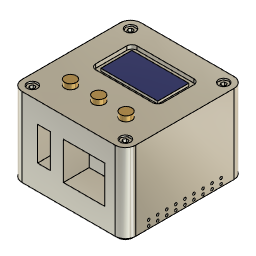
NanoPi v2 v1 (Autodesk Fusion 360 design; units mm, degrees)
Autodesk Fusion 360 part; units mm, degrees
sketch "草图1" plane through (0, 0, 0) normal (0, 0, 1) x (1, 0, 0)
  line L0 (4, 0) -> (40, 0)
  line L1 (44, 4) -> (44, 42)
  line L2 (40, 46) -> (4, 46)
  line L3 (0, 42) -> (0, 4)
  arc A0 (4, 46) -> (0, 42) centre (4, 42) ccw
  arc A1 (44, 42) -> (40, 46) centre (40, 42) ccw
  arc A2 (40, 0) -> (44, 4) centre (40, 4) ccw
  arc A3 (0, 4) -> (4, 0) centre (4, 4) ccw
  point P0 (44, 0)
  point P1 (0, 46)
  dimension "d1" = 44
  dimension "d2" = 46
  dimension "d3" = 4
  dimension "d4" = 4
  dimension "d5" = 4
  dimension "d6" = 4
  constraint horizontal L0
  constraint vertical L1
  constraint horizontal L2
  constraint vertical L3
  constraint coincident P1 L2
  constraint coincident P1 L3
  constraint tangent L2 A0
  constraint tangent L3 A0
  constraint tangent L2 A1
  constraint tangent L1 A1
  constraint coincident P0 L1
  constraint coincident P0 L0
  constraint tangent L1 A2
  constraint tangent L0 A2
  constraint coincident origin L3
  constraint coincident origin L0
  constraint tangent L3 A3
  constraint tangent L0 A3
  measures "d1" distance of origin P0
  measures "d2" distance of origin P1
  measures "d3" radius of A0
  measures "d4" radius of A1
  measures "d5" radius of A2
  measures "d6" radius of A3
extrude "拉伸1" add sketch "草图1" along normal blind 30.5 makes body 1
sketch "草图2" plane through (0, 0, 30.5) normal (0, 0, 1) x (-1, 0, 0)
  arc A0 (0, -4) -> (-4, 0) centre (-4, -4) ccw
  line L0 (-4, 0) -> (-40, 0)
  arc A1 (-40, 0) -> (-44, -4) centre (-40, -4) ccw
  line L1 (-44, -4) -> (-44, -42)
  arc A2 (-44, -42) -> (-40, -46) centre (-40, -42) ccw
  line L2 (-40, -46) -> (-4, -46)
  arc A3 (-4, -46) -> (0, -42) centre (-4, -42) ccw
  line L3 (0, -42) -> (0, -4)
  line L4 (-11, -37.5) -> (-33, -37.5)
  line L5 (-35, -35.5) -> (-35, -23.5)
  line L6 (-33, -21.5) -> (-11, -21.5)
  line L7 (-9, -23.5) -> (-9, -35.5)
  arc A4 (-11, -37.5) -> (-9, -35.5) centre (-11, -35.5) ccw
  arc A5 (-35, -35.5) -> (-33, -37.5) centre (-33, -35.5) ccw
  arc A6 (-33, -21.5) -> (-35, -23.5) centre (-33, -23.5) ccw
  arc A7 (-9, -23.5) -> (-11, -21.5) centre (-11, -23.5) ccw
  point P0 (-9, -37.5)
  point P1 (-35, -37.5)
  point P2 (-9, -21.5)
  dimension "d9" = 26
  dimension "d10" = 16
  dimension "d11" = 8.5
  dimension "d12" = 9
  dimension "d13" = 2
  dimension "d14" = 2
  dimension "d15" = 2
  dimension "d16" = 2
  constraint horizontal L4
  constraint vertical L5
  constraint horizontal L6
  constraint vertical L7
  constraint coincident P0 L4
  constraint coincident P0 L7
  constraint tangent L4 A4
  constraint tangent L7 A4
  constraint coincident P1 L4
  constraint coincident P1 L5
  constraint tangent L4 A5
  constraint tangent L5 A5
  constraint tangent L5 A6
  constraint tangent L6 A6
  constraint coincident P2 L7
  constraint coincident P2 L6
  constraint tangent L7 A7
  constraint tangent L6 A7
  measures "d9" distance of P0 P1
  measures "d10" distance of P0 P2
  measures "d11" distance of L2 L4
  measures "d12" distance of L3 L7
  measures "d13" radius of A4
  measures "d14" radius of A5
  measures "d15" radius of A6
  measures "d16" radius of A7
extrude "拉伸2" cut sketch "草图2" against normal blind 1.5 contours L4 L5 L6 L7 A4 A5 A6 A7 bodies 1
sketch "草图3" plane through (0, 0, 29) normal (0, 0, 1) x (-1, 0, 0)
  arc A0 (-11, -37.5) -> (-9, -35.5) centre (-11, -35.5) ccw
  line L0 (-9, -35.5) -> (-9, -23.5)
  arc A1 (-9, -23.5) -> (-11, -21.5) centre (-11, -23.5) ccw
  line L1 (-11, -21.5) -> (-33, -21.5)
  arc A2 (-33, -21.5) -> (-35, -23.5) centre (-33, -23.5) ccw
  line L2 (-35, -23.5) -> (-35, -35.5)
  arc A3 (-35, -35.5) -> (-33, -37.5) centre (-33, -35.5) ccw
  line L3 (-33, -37.5) -> (-11, -37.5)
  line L4 (-11, -35.5) -> (-33, -35.5)
  line L5 (-33, -35.5) -> (-33, -23.5)
  line L6 (-33, -23.5) -> (-11, -23.5)
  line L7 (-11, -23.5) -> (-11, -35.5)
  constraint horizontal L4
  constraint vertical L5
  constraint horizontal L6
  constraint vertical L7
  constraint coincident A2.centre L5.end
  constraint coincident A0.centre L4.start
extrude "拉伸3" add sketch "草图3" along normal blind 1 contours L4 L5 L6 L7 bodies 1
sketch "草图4" plane through (0, 0, 30.5) normal (0, 0, 1) x (-1, 0, 0)
  line L0 (-9, -23.5) -> (-9, -35.5)
  arc A0 (-11, -37.5) -> (-9, -35.5) centre (-11, -35.5) ccw
  line L1 (-11, -37.5) -> (-33, -37.5)
  arc A1 (-35, -35.5) -> (-33, -37.5) centre (-33, -35.5) ccw
  line L2 (-35, -35.5) -> (-35, -23.5)
  arc A2 (-33, -21.5) -> (-35, -23.5) centre (-33, -23.5) ccw
  line L3 (-33, -21.5) -> (-11, -21.5)
  arc A3 (-9, -23.5) -> (-11, -21.5) centre (-11, -23.5) ccw
  arc A4 (0, -4) -> (-4, 0) centre (-4, -4) ccw
  line L4 (-4, 0) -> (-40, 0)
  arc A5 (-40, 0) -> (-44, -4) centre (-40, -4) ccw
  line L5 (-44, -4) -> (-44, -42)
  arc A6 (-44, -42) -> (-40, -46) centre (-40, -42) ccw
  line L6 (-40, -46) -> (-4, -46)
  arc A7 (-4, -46) -> (0, -42) centre (-4, -42) ccw
  line L7 (0, -42) -> (0, -4)
  circle A8 centre (-4, -42) radius 2
  circle A9 centre (-40, -42) radius 2
  circle A10 centre (-4, -4) radius 2
  circle A11 centre (-40, -4) radius 2
  dimension "d21" = 4
  dimension "d22" = 4
  dimension "d23" = 4
  dimension "d24" = 4
  constraint concentric A7 A8
  constraint concentric A6 A9
  constraint concentric A4 A10
  constraint concentric A5 A11
  measures "d21" diameter of A8
  measures "d22" diameter of A9
  measures "d23" diameter of A10
  measures "d24" diameter of A11
extrude "拉伸4" cut sketch "草图4" against normal blind 2 contours A8 | A9 | A10 | A11 bodies 1
sketch "草图5" plane through (0, 0, 28.5) normal (0, 0, 1) x (-1, 0, 0)
  circle A0 centre (-4, -42) radius 2
  line L0 (-4.9596, -43.7548) -> (-2.9601, -43.7084)
  line L1 (-2.9601, -43.7084) -> (-2.0005, -41.9537)
  line L2 (-2.0005, -41.9537) -> (-3.0404, -40.2452)
  line L3 (-3.0404, -40.2452) -> (-5.0399, -40.2916)
  line L4 (-5.0399, -40.2916) -> (-5.9995, -42.0463)
  line L5 (-5.9995, -42.0463) -> (-4.9596, -43.7548)
  line L6 (-4.5137, -42.8579) -> (-3.5139, -42.8739)
  line L7 (-3.5139, -42.8739) -> (-3.0001, -42.016)
  line L8 (-3.0001, -42.016) -> (-3.4863, -41.1421)
  line L9 (-3.4863, -41.1421) -> (-4.4861, -41.1261)
  line L10 (-4.4861, -41.1261) -> (-4.9999, -41.984)
  line L11 (-4.9999, -41.984) -> (-4.5137, -42.8579)
  line L12 (-41.835, -42.7954) -> (-40.2287, -43.9869)
  line L13 (-40.2287, -43.9869) -> (-38.3937, -43.1915)
  line L14 (-38.3937, -43.1915) -> (-38.165, -41.2046)
  line L15 (-38.165, -41.2046) -> (-39.7713, -40.0131)
  line L16 (-39.7713, -40.0131) -> (-41.6063, -40.8085)
  line L17 (-41.6063, -40.8085) -> (-41.835, -42.7954)
  line L18 (-41, -42) -> (-40.5, -42.866)
  line L19 (-40.5, -42.866) -> (-39.5, -42.866)
  line L20 (-39.5, -42.866) -> (-39, -42)
  line L21 (-39, -42) -> (-39.5, -41.134)
  line L22 (-39.5, -41.134) -> (-40.5, -41.134)
  line L23 (-40.5, -41.134) -> (-41, -42)
  line L24 (-6, -4) -> (-5, -5.7321)
  line L25 (-5, -5.7321) -> (-3, -5.7321)
  line L26 (-3, -5.7321) -> (-2, -4)
  line L27 (-2, -4) -> (-3, -2.2679)
  line L28 (-3, -2.2679) -> (-5, -2.2679)
  line L29 (-5, -2.2679) -> (-6, -4)
  line L30 (-5, -4) -> (-4.5, -4.866)
  line L31 (-4.5, -4.866) -> (-3.5, -4.866)
  line L32 (-3.5, -4.866) -> (-3, -4)
  line L33 (-3, -4) -> (-3.5, -3.134)
  line L34 (-3.5, -3.134) -> (-4.5, -3.134)
  line L35 (-4.5, -3.134) -> (-5, -4)
  line L36 (-42, -4) -> (-41, -5.7321)
  line L37 (-41, -5.7321) -> (-39, -5.7321)
  line L38 (-39, -5.7321) -> (-38, -4)
  line L39 (-38, -4) -> (-39, -2.2679)
  line L40 (-39, -2.2679) -> (-41, -2.2679)
  line L41 (-41, -2.2679) -> (-42, -4)
  line L42 (-41, -4) -> (-40.5, -4.866)
  line L43 (-40.5, -4.866) -> (-39.5, -4.866)
  line L44 (-39.5, -4.866) -> (-39, -4)
  line L45 (-39, -4) -> (-39.5, -3.134)
  line L46 (-39.5, -3.134) -> (-40.5, -3.134)
  line L47 (-40.5, -3.134) -> (-41, -4)
  point P0 (-4, -42)
  point P1 (-4, -42)
  point P2 (-40, -42)
  point P3 (-40, -42)
  point P4 (-4, -4)
  point P5 (-4, -4)
  point P6 (-40, -4)
  point P7 (-40, -4)
  dimension "d27" = 1
  dimension "d28" = 2
  dimension "d29" = 1
  dimension "d30" = 2
  dimension "d31" = 1
  dimension "d32" = 2
  dimension "d33" = 1
  constraint coincident A0 L0.start
  constraint coincident P0 A0.centre
  constraint coincident P1 P0
  constraint coincident P3 P2
  constraint coincident P5 P4
  constraint coincident P7 P6
  measures "d27" distance of L6.start P1
  measures "d28" distance of L12.start P3
  measures "d29" distance of L18.start P3
  measures "d30" distance of L24.start P5
  measures "d31" distance of L30.start P5
  measures "d32" distance of L36.start P7
  measures "d33" distance of L42.start P7
extrude "拉伸5" add sketch "草图5" along normal blind 1.5 separate body contours L0 L1 L2 L3 L4 L5 | L12 L13 L14 L15 L16 L17 | L24 L25 L26 L27 L28 L29 | L36 L37 L38 L39 L40 L41 makes body 2 at (40.6259, 40.6519, 28.5) makes body 3 at (5.3333, 4.5774, 28.5) makes body 4 at (3.8112, 43.4457, 28.5) makes body 5 at (38.6667, 4.5774, 28.5)
sketch "草图6" plane through (0, 0, 30.5) normal (0, 0, 1) x (-1, 0, 0)
  circle A0 centre (-40, -42) radius 2
  circle A1 centre (-40, -4) radius 2
  circle A2 centre (-4, -42) radius 2
  circle A3 centre (-4, -4) radius 2
  line L0 (-9, -23.5) -> (-9, -35.5)
  arc A4 (-11, -37.5) -> (-9, -35.5) centre (-11, -35.5) ccw
  line L1 (-11, -37.5) -> (-33, -37.5)
  arc A5 (-35, -35.5) -> (-33, -37.5) centre (-33, -35.5) ccw
  line L2 (-35, -35.5) -> (-35, -23.5)
  arc A6 (-33, -21.5) -> (-35, -23.5) centre (-33, -23.5) ccw
  line L3 (-33, -21.5) -> (-11, -21.5)
  arc A7 (-9, -23.5) -> (-11, -21.5) centre (-11, -23.5) ccw
  arc A8 (0, -4) -> (-4, 0) centre (-4, -4) ccw
  line L4 (-4, 0) -> (-40, 0)
  arc A9 (-40, 0) -> (-44, -4) centre (-40, -4) ccw
  line L5 (-44, -4) -> (-44, -42)
  arc A10 (-44, -42) -> (-40, -46) centre (-40, -42) ccw
  line L6 (-40, -46) -> (-4, -46)
  arc A11 (-4, -46) -> (0, -42) centre (-4, -42) ccw
  line L7 (0, -42) -> (0, -4)
  circle A12 centre (-11.25, -11.5) radius 2.25
  circle A13 centre (-22, -11.6939) radius 2.25
  circle A14 centre (-32.75, -11.5) radius 2.25
  line L8 (-22, -37.5) -> (-22, -11.6939) construction
  dimension "d36" = 4.5
  dimension "d37" = 4.5
  dimension "d38" = 4.5
  dimension "d39" = 10
  dimension "d40" = 10
  constraint tangent L0 A12
  constraint tangent L2 A14
  constraint midpoint L1 L8.start
  constraint perpendicular L3 L8
  constraint coincident A13.centre L8.end
  measures "d36" diameter of A12
  measures "d37" diameter of A13
  measures "d38" diameter of A14
  measures "d39" distance of L3 A12.centre
  measures "d40" distance of L3 A14.centre
extrude "拉伸6" add sketch "草图6" along normal blind 2 contours A12 | A13 | A14 bodies 1
sketch "草图7" plane through (44, 0, 0) normal (1, 0, 0) x (0, 1, 0)
  line L0 (4, 0) -> (42, 0)
  line L1 (42, 0) -> (42, 30.5)
  line L2 (42, 30.5) -> (4, 30.5)
  line L3 (4, 30.5) -> (4, 0)
  circle A0 centre (37, 1) radius 0.5
  circle A1 centre (33.5, 1) radius 0.5
  circle A2 centre (30, 1) radius 0.5
  circle A3 centre (26.5, 1) radius 0.5
  circle A4 centre (23, 1) radius 0.5
  circle A5 centre (19.5, 1) radius 0.5
  circle A6 centre (16, 1) radius 0.5
  circle A7 centre (12.5, 1) radius 0.5
  circle A8 centre (9, 1) radius 0.5
  circle A9 centre (37, 3) radius 0.5
  circle A10 centre (33.5, 3) radius 0.5
  circle A11 centre (30, 3) radius 0.5
  circle A12 centre (26.5, 3) radius 0.5
  circle A13 centre (23, 3) radius 0.5
  circle A14 centre (19.5, 3) radius 0.5
  circle A15 centre (16, 3) radius 0.5
  circle A16 centre (12.5, 3) radius 0.5
  circle A17 centre (9, 3) radius 0.5
  dimension "d43" = 1
  dimension "d46" = -28
  dimension "d47" = 2
  measures "d43" diameter of A0
extrude "拉伸7" cut sketch "草图7" against normal blind 3 contours A0 | A1 | A2 | A3 | A4 | A5 | A6 | A7 | A8 | A9 | A10 | A11 | A12 | A13 | A14 | A15 | A16 | A17 bodies 1
sketch "草图8" plane through (0, 0, 0) normal (-1, 0, 0) x (0, -1, 0)
  line L0 (-42, 0) -> (-4, 0)
  line L1 (-4, 0) -> (-4, 30.5)
  line L2 (-4, 30.5) -> (-42, 30.5)
  line L3 (-42, 30.5) -> (-42, 0)
  circle A0 centre (-9, 1.0003) radius 0.5
  circle A1 centre (-12.5, 1.0003) radius 0.5
  circle A2 centre (-16, 1.0003) radius 0.5
  circle A3 centre (-19.5, 1.0003) radius 0.5
  circle A4 centre (-23, 1.0003) radius 0.5
  circle A5 centre (-26.5, 1.0003) radius 0.5
  circle A6 centre (-30, 1.0003) radius 0.5
  circle A7 centre (-33.5, 1.0003) radius 0.5
  circle A8 centre (-37, 1.0003) radius 0.5
  circle A9 centre (-9, 3.0003) radius 0.5
  circle A10 centre (-12.5, 3.0003) radius 0.5
  circle A11 centre (-16, 3.0003) radius 0.5
  circle A12 centre (-19.5, 3.0003) radius 0.5
  circle A13 centre (-23, 3.0003) radius 0.5
  circle A14 centre (-26.5, 3.0003) radius 0.5
  circle A15 centre (-30, 3.0003) radius 0.5
  circle A16 centre (-33.5, 3.0003) radius 0.5
  circle A17 centre (-37, 3.0003) radius 0.5
  dimension "d50" = 1
  dimension "d51" = 5
  dimension "d54" = -28
  dimension "d55" = 2
  measures "d50" diameter of A0
  measures "d51" distance of L1 A0.centre
extrude "拉伸8" cut sketch "草图8" against normal blind 3 contours A0 | A1 | A2 | A3 | A4 | A5 | A6 | A7 | A8 | A9 | A10 | A11 | A12 | A13 | A14 | A15 | A16 | A17 bodies 1
sketch "草图9" plane through (0, 0, 0) normal (0, 0, -1) x (1, 0, 0)
  arc A0 (4, 0) -> (0, -4) centre (4, -4) ccw
  line L0 (0, -4) -> (0, -42)
  arc A1 (0, -42) -> (4, -46) centre (4, -42) ccw
  line L1 (4, -46) -> (40, -46)
  arc A2 (40, -46) -> (44, -42) centre (40, -42) ccw
  line L2 (44, -42) -> (44, -4)
  arc A3 (44, -4) -> (40, 0) centre (40, -4) ccw
  line L3 (40, 0) -> (4, 0)
  circle A4 centre (40, -42) radius 3
  circle A5 centre (4, -42) radius 3
  circle A6 centre (40, -4) radius 3
  circle A7 centre (4, -4) radius 3
  line L4 (41, -38.127) -> (41, -7.873)
  line L5 (36.127, -43) -> (7.873, -43)
  line L6 (3, -38.127) -> (3, -7.873)
  line L7 (36.127, -3) -> (7.873, -3)
  arc A8 (36.127, -3) -> (41, -7.873) centre (40, -4) ccw
  arc A9 (3, -7.873) -> (7.873, -3) centre (4, -4) ccw
  arc A10 (4, 0) -> (0, -4) centre (4, -4) ccw
  arc A11 (7.873, -43) -> (3, -38.127) centre (4, -42) ccw
  arc A12 (0, -42) -> (4, -46) centre (4, -42) ccw
  arc A13 (41, -38.127) -> (36.127, -43) centre (40, -42) ccw
  arc A14 (40, -46) -> (44, -42) centre (40, -42) ccw
  line L8 (35, -42) -> (30, -42)
  line L9 (30, -42) -> (30, -41)
  line L10 (30, -41) -> (35, -41)
  line L11 (35, -41) -> (35, -42)
  line L12 (28, -41) -> (28, -42)
  line L13 (28, -42) -> (23, -42)
  line L14 (23, -41) -> (28, -41)
  line L15 (23, -42) -> (23, -41)
  line L16 (21, -41) -> (21, -42)
  line L17 (21, -42) -> (16, -42)
  line L18 (16, -41) -> (21, -41)
  line L19 (16, -42) -> (16, -41)
  line L20 (14, -41) -> (14, -42)
  line L21 (14, -42) -> (9, -42)
  line L22 (9, -41) -> (14, -41)
  line L23 (9, -42) -> (9, -41)
  line L24 (35, -38.3571) -> (35, -39.3571)
  line L25 (35, -39.3571) -> (30, -39.3571)
  line L26 (30, -38.3571) -> (35, -38.3571)
  line L27 (30, -39.3571) -> (30, -38.3571)
  line L28 (28, -38.3571) -> (28, -39.3571)
  line L29 (28, -39.3571) -> (23, -39.3571)
  line L30 (23, -38.3571) -> (28, -38.3571)
  line L31 (23, -39.3571) -> (23, -38.3571)
  line L32 (21, -38.3571) -> (21, -39.3571)
  line L33 (21, -39.3571) -> (16, -39.3571)
  line L34 (16, -38.3571) -> (21, -38.3571)
  line L35 (16, -39.3571) -> (16, -38.3571)
  line L36 (14, -38.3571) -> (14, -39.3571)
  line L37 (14, -39.3571) -> (9, -39.3571)
  line L38 (9, -38.3571) -> (14, -38.3571)
  line L39 (9, -39.3571) -> (9, -38.3571)
  line L40 (35, -35.7143) -> (35, -36.7143)
  line L41 (35, -36.7143) -> (30, -36.7143)
  line L42 (30, -35.7143) -> (35, -35.7143)
  line L43 (30, -36.7143) -> (30, -35.7143)
  line L44 (28, -35.7143) -> (28, -36.7143)
  line L45 (28, -36.7143) -> (23, -36.7143)
  line L46 (23, -35.7143) -> (28, -35.7143)
  line L47 (23, -36.7143) -> (23, -35.7143)
  line L48 (21, -35.7143) -> (21, -36.7143)
  line L49 (21, -36.7143) -> (16, -36.7143)
  line L50 (16, -35.7143) -> (21, -35.7143)
  line L51 (16, -36.7143) -> (16, -35.7143)
  line L52 (14, -35.7143) -> (14, -36.7143)
  line L53 (14, -36.7143) -> (9, -36.7143)
  line L54 (9, -35.7143) -> (14, -35.7143)
  line L55 (9, -36.7143) -> (9, -35.7143)
  line L56 (35, -33.0714) -> (35, -34.0714)
  line L57 (35, -34.0714) -> (30, -34.0714)
  line L58 (30, -33.0714) -> (35, -33.0714)
  line L59 (30, -34.0714) -> (30, -33.0714)
  line L60 (28, -33.0714) -> (28, -34.0714)
  line L61 (28, -34.0714) -> (23, -34.0714)
  line L62 (23, -33.0714) -> (28, -33.0714)
  line L63 (23, -34.0714) -> (23, -33.0714)
  line L64 (21, -33.0714) -> (21, -34.0714)
  line L65 (21, -34.0714) -> (16, -34.0714)
  line L66 (16, -33.0714) -> (21, -33.0714)
  line L67 (16, -34.0714) -> (16, -33.0714)
  line L68 (14, -33.0714) -> (14, -34.0714)
  line L69 (14, -34.0714) -> (9, -34.0714)
  line L70 (9, -33.0714) -> (14, -33.0714)
  line L71 (9, -34.0714) -> (9, -33.0714)
  line L72 (35, -30.4286) -> (35, -31.4286)
  line L73 (35, -31.4286) -> (30, -31.4286)
  line L74 (30, -30.4286) -> (35, -30.4286)
  line L75 (30, -31.4286) -> (30, -30.4286)
  line L76 (28, -30.4286) -> (28, -31.4286)
  line L77 (28, -31.4286) -> (23, -31.4286)
  line L78 (23, -30.4286) -> (28, -30.4286)
  line L79 (23, -31.4286) -> (23, -30.4286)
  line L80 (21, -30.4286) -> (21, -31.4286)
  line L81 (21, -31.4286) -> (16, -31.4286)
  line L82 (16, -30.4286) -> (21, -30.4286)
  line L83 (16, -31.4286) -> (16, -30.4286)
  line L84 (14, -30.4286) -> (14, -31.4286)
  line L85 (14, -31.4286) -> (9, -31.4286)
  line L86 (9, -30.4286) -> (14, -30.4286)
  line L87 (9, -31.4286) -> (9, -30.4286)
  line L88 (35, -27.7857) -> (35, -28.7857)
  line L89 (35, -28.7857) -> (30, -28.7857)
  line L90 (30, -27.7857) -> (35, -27.7857)
  line L91 (30, -28.7857) -> (30, -27.7857)
  line L92 (28, -27.7857) -> (28, -28.7857)
  line L93 (28, -28.7857) -> (23, -28.7857)
  line L94 (23, -27.7857) -> (28, -27.7857)
  line L95 (23, -28.7857) -> (23, -27.7857)
  line L96 (21, -27.7857) -> (21, -28.7857)
  line L97 (21, -28.7857) -> (16, -28.7857)
  line L98 (16, -27.7857) -> (21, -27.7857)
  line L99 (16, -28.7857) -> (16, -27.7857)
  line L100 (14, -27.7857) -> (14, -28.7857)
  line L101 (14, -28.7857) -> (9, -28.7857)
  line L102 (9, -27.7857) -> (14, -27.7857)
  line L103 (9, -28.7857) -> (9, -27.7857)
  line L104 (35, -25.1429) -> (35, -26.1429)
  line L105 (35, -26.1429) -> (30, -26.1429)
  line L106 (30, -25.1429) -> (35, -25.1429)
  line L107 (30, -26.1429) -> (30, -25.1429)
  line L108 (28, -25.1429) -> (28, -26.1429)
  line L109 (28, -26.1429) -> (23, -26.1429)
  line L110 (23, -25.1429) -> (28, -25.1429)
  line L111 (23, -26.1429) -> (23, -25.1429)
  line L112 (21, -25.1429) -> (21, -26.1429)
  line L113 (21, -26.1429) -> (16, -26.1429)
  line L114 (16, -25.1429) -> (21, -25.1429)
  line L115 (16, -26.1429) -> (16, -25.1429)
  line L116 (14, -25.1429) -> (14, -26.1429)
  line L117 (14, -26.1429) -> (9, -26.1429)
  line L118 (9, -25.1429) -> (14, -25.1429)
  line L119 (9, -26.1429) -> (9, -25.1429)
  line L120 (35, -22.5) -> (35, -23.5)
  line L121 (35, -23.5) -> (30, -23.5)
  line L122 (30, -22.5) -> (35, -22.5)
  line L123 (30, -23.5) -> (30, -22.5)
  line L124 (28, -22.5) -> (28, -23.5)
  line L125 (28, -23.5) -> (23, -23.5)
  line L126 (23, -22.5) -> (28, -22.5)
  line L127 (23, -23.5) -> (23, -22.5)
  line L128 (21, -22.5) -> (21, -23.5)
  line L129 (21, -23.5) -> (16, -23.5)
  line L130 (16, -22.5) -> (21, -22.5)
  line L131 (16, -23.5) -> (16, -22.5)
  line L132 (14, -22.5) -> (14, -23.5)
  line L133 (14, -23.5) -> (9, -23.5)
  line L134 (9, -22.5) -> (14, -22.5)
  line L135 (9, -23.5) -> (9, -22.5)
  line L136 (35, -19.8571) -> (35, -20.8571)
  line L137 (35, -20.8571) -> (30, -20.8571)
  line L138 (30, -19.8571) -> (35, -19.8571)
  line L139 (30, -20.8571) -> (30, -19.8571)
  line L140 (28, -19.8571) -> (28, -20.8571)
  line L141 (28, -20.8571) -> (23, -20.8571)
  line L142 (23, -19.8571) -> (28, -19.8571)
  line L143 (23, -20.8571) -> (23, -19.8571)
  line L144 (21, -19.8571) -> (21, -20.8571)
  line L145 (21, -20.8571) -> (16, -20.8571)
  line L146 (16, -19.8571) -> (21, -19.8571)
  line L147 (16, -20.8571) -> (16, -19.8571)
  line L148 (14, -19.8571) -> (14, -20.8571)
  line L149 (14, -20.8571) -> (9, -20.8571)
  line L150 (9, -19.8571) -> (14, -19.8571)
  line L151 (9, -20.8571) -> (9, -19.8571)
  line L152 (35, -17.2143) -> (35, -18.2143)
  line L153 (35, -18.2143) -> (30, -18.2143)
  line L154 (30, -17.2143) -> (35, -17.2143)
  line L155 (30, -18.2143) -> (30, -17.2143)
  line L156 (28, -17.2143) -> (28, -18.2143)
  line L157 (28, -18.2143) -> (23, -18.2143)
  line L158 (23, -17.2143) -> (28, -17.2143)
  line L159 (23, -18.2143) -> (23, -17.2143)
  line L160 (21, -17.2143) -> (21, -18.2143)
  line L161 (21, -18.2143) -> (16, -18.2143)
  line L162 (16, -17.2143) -> (21, -17.2143)
  line L163 (16, -18.2143) -> (16, -17.2143)
  line L164 (14, -17.2143) -> (14, -18.2143)
  line L165 (14, -18.2143) -> (9, -18.2143)
  line L166 (9, -17.2143) -> (14, -17.2143)
  line L167 (9, -18.2143) -> (9, -17.2143)
  line L168 (35, -14.5714) -> (35, -15.5714)
  line L169 (35, -15.5714) -> (30, -15.5714)
  line L170 (30, -14.5714) -> (35, -14.5714)
  line L171 (30, -15.5714) -> (30, -14.5714)
  line L172 (28, -14.5714) -> (28, -15.5714)
  line L173 (28, -15.5714) -> (23, -15.5714)
  line L174 (23, -14.5714) -> (28, -14.5714)
  line L175 (23, -15.5714) -> (23, -14.5714)
  line L176 (21, -14.5714) -> (21, -15.5714)
  line L177 (21, -15.5714) -> (16, -15.5714)
  line L178 (16, -14.5714) -> (21, -14.5714)
  line L179 (16, -15.5714) -> (16, -14.5714)
  line L180 (14, -14.5714) -> (14, -15.5714)
  line L181 (14, -15.5714) -> (9, -15.5714)
  line L182 (9, -14.5714) -> (14, -14.5714)
  line L183 (9, -15.5714) -> (9, -14.5714)
  line L184 (35, -11.9286) -> (35, -12.9286)
  line L185 (35, -12.9286) -> (30, -12.9286)
  line L186 (30, -11.9286) -> (35, -11.9286)
  line L187 (30, -12.9286) -> (30, -11.9286)
  line L188 (28, -11.9286) -> (28, -12.9286)
  line L189 (28, -12.9286) -> (23, -12.9286)
  line L190 (23, -11.9286) -> (28, -11.9286)
  line L191 (23, -12.9286) -> (23, -11.9286)
  line L192 (21, -11.9286) -> (21, -12.9286)
  line L193 (21, -12.9286) -> (16, -12.9286)
  line L194 (16, -11.9286) -> (21, -11.9286)
  line L195 (16, -12.9286) -> (16, -11.9286)
  line L196 (14, -11.9286) -> (14, -12.9286)
  line L197 (14, -12.9286) -> (9, -12.9286)
  line L198 (9, -11.9286) -> (14, -11.9286)
  line L199 (9, -12.9286) -> (9, -11.9286)
  line L200 (35, -9.2857) -> (35, -10.2857)
  line L201 (35, -10.2857) -> (30, -10.2857)
  line L202 (30, -9.2857) -> (35, -9.2857)
  line L203 (30, -10.2857) -> (30, -9.2857)
  line L204 (28, -9.2857) -> (28, -10.2857)
  line L205 (28, -10.2857) -> (23, -10.2857)
  line L206 (23, -9.2857) -> (28, -9.2857)
  line L207 (23, -10.2857) -> (23, -9.2857)
  line L208 (21, -9.2857) -> (21, -10.2857)
  line L209 (21, -10.2857) -> (16, -10.2857)
  line L210 (16, -9.2857) -> (21, -9.2857)
  line L211 (16, -10.2857) -> (16, -9.2857)
  line L212 (14, -9.2857) -> (14, -10.2857)
  line L213 (14, -10.2857) -> (9, -10.2857)
  line L214 (9, -9.2857) -> (14, -9.2857)
  line L215 (9, -10.2857) -> (9, -9.2857)
  line L216 (35, -6.6429) -> (35, -7.6429)
  line L217 (35, -7.6429) -> (30, -7.6429)
  line L218 (30, -6.6429) -> (35, -6.6429)
  line L219 (30, -7.6429) -> (30, -6.6429)
  line L220 (28, -6.6429) -> (28, -7.6429)
  line L221 (28, -7.6429) -> (23, -7.6429)
  line L222 (23, -6.6429) -> (28, -6.6429)
  line L223 (23, -7.6429) -> (23, -6.6429)
  line L224 (21, -6.6429) -> (21, -7.6429)
  line L225 (21, -7.6429) -> (16, -7.6429)
  line L226 (16, -6.6429) -> (21, -6.6429)
  line L227 (16, -7.6429) -> (16, -6.6429)
  line L228 (14, -6.6429) -> (14, -7.6429)
  line L229 (14, -7.6429) -> (9, -7.6429)
  line L230 (9, -6.6429) -> (14, -6.6429)
  line L231 (9, -7.6429) -> (9, -6.6429)
  line L232 (35, -4) -> (35, -5)
  line L233 (35, -5) -> (30, -5)
  line L234 (30, -4) -> (35, -4)
  line L235 (30, -5) -> (30, -4)
  line L236 (28, -4) -> (28, -5)
  line L237 (28, -5) -> (23, -5)
  line L238 (23, -4) -> (28, -4)
  line L239 (23, -5) -> (23, -4)
  line L240 (21, -4) -> (21, -5)
  line L241 (21, -5) -> (16, -5)
  line L242 (16, -4) -> (21, -4)
  line L243 (16, -5) -> (16, -4)
  line L244 (14, -4) -> (14, -5)
  line L245 (14, -5) -> (9, -5)
  line L246 (9, -4) -> (14, -4)
  line L247 (9, -5) -> (9, -4)
  line L248 (36.3819, -35.7143) -> (40.3682, -35.7143)
  line L249 (40.3682, -35.7143) -> (40.3682, -36.6815)
  line L250 (40.3682, -36.6815) -> (36.3819, -36.6815)
  line L251 (35, -36.6815) -> (35, -35.7143)
  line L252 (36.3819, -36.6815) -> (36.3819, -35.7143)
  line L253 (36.3819, -33.9815) -> (36.3819, -33.0143)
  line L254 (36.3819, -33.0143) -> (40.3682, -33.0143)
  line L255 (40.3682, -33.9815) -> (36.3819, -33.9815)
  line L256 (40.3682, -33.0143) -> (40.3682, -33.9815)
  line L257 (36.3819, -31.2815) -> (36.3819, -30.3143)
  line L258 (36.3819, -30.3143) -> (40.3682, -30.3143)
  line L259 (40.3682, -31.2815) -> (36.3819, -31.2815)
  line L260 (40.3682, -30.3143) -> (40.3682, -31.2815)
  line L261 (36.3819, -28.5815) -> (36.3819, -27.6143)
  line L262 (36.3819, -27.6143) -> (40.3682, -27.6143)
  line L263 (40.3682, -28.5815) -> (36.3819, -28.5815)
  line L264 (40.3682, -27.6143) -> (40.3682, -28.5815)
  line L265 (36.3819, -25.8815) -> (36.3819, -24.9143)
  line L266 (36.3819, -24.9143) -> (40.3682, -24.9143)
  line L267 (40.3682, -25.8815) -> (36.3819, -25.8815)
  line L268 (40.3682, -24.9143) -> (40.3682, -25.8815)
  line L269 (36.3819, -23.1815) -> (36.3819, -22.2143)
  line L270 (36.3819, -22.2143) -> (40.3682, -22.2143)
  line L271 (40.3682, -23.1815) -> (36.3819, -23.1815)
  line L272 (40.3682, -22.2143) -> (40.3682, -23.1815)
  line L273 (36.3819, -20.4815) -> (36.3819, -19.5143)
  line L274 (36.3819, -19.5143) -> (40.3682, -19.5143)
  line L275 (40.3682, -20.4815) -> (36.3819, -20.4815)
  line L276 (40.3682, -19.5143) -> (40.3682, -20.4815)
  line L277 (36.3819, -17.7815) -> (36.3819, -16.8143)
  line L278 (36.3819, -16.8143) -> (40.3682, -16.8143)
  line L279 (40.3682, -17.7815) -> (36.3819, -17.7815)
  line L280 (40.3682, -16.8143) -> (40.3682, -17.7815)
  line L281 (36.3819, -15.0815) -> (36.3819, -14.1143)
  line L282 (36.3819, -14.1143) -> (40.3682, -14.1143)
  line L283 (40.3682, -15.0815) -> (36.3819, -15.0815)
  line L284 (40.3682, -14.1143) -> (40.3682, -15.0815)
  line L285 (36.3819, -12.3815) -> (36.3819, -11.4143)
  line L286 (36.3819, -11.4143) -> (40.3682, -11.4143)
  line L287 (40.3682, -12.3815) -> (36.3819, -12.3815)
  line L288 (40.3682, -11.4143) -> (40.3682, -12.3815)
  line L289 (36.3819, -9.6815) -> (36.3819, -8.7143)
  line L290 (36.3819, -8.7143) -> (40.3682, -8.7143)
  line L291 (40.3682, -9.6815) -> (36.3819, -9.6815)
  line L292 (40.3682, -8.7143) -> (40.3682, -9.6815)
  line L293 (7.8388, -36.6694) -> (3.5388, -36.6694)
  line L294 (3.5388, -36.6694) -> (3.5388, -35.6694)
  line L295 (3.5388, -35.6694) -> (7.8388, -35.6694)
  line L296 (7.8388, -35.6694) -> (7.8388, -36.6694)
  line L297 (7.8388, -33.9694) -> (3.5388, -33.9694)
  line L298 (7.8388, -32.9694) -> (7.8388, -33.9694)
  line L299 (3.5388, -32.9694) -> (7.8388, -32.9694)
  line L300 (3.5388, -33.9694) -> (3.5388, -32.9694)
  line L301 (7.8388, -31.2694) -> (3.5388, -31.2694)
  line L302 (7.8388, -30.2694) -> (7.8388, -31.2694)
  line L303 (3.5388, -30.2694) -> (7.8388, -30.2694)
  line L304 (3.5388, -31.2694) -> (3.5388, -30.2694)
  line L305 (7.8388, -28.5694) -> (3.5388, -28.5694)
  line L306 (7.8388, -27.5694) -> (7.8388, -28.5694)
  line L307 (3.5388, -27.5694) -> (7.8388, -27.5694)
  line L308 (3.5388, -28.5694) -> (3.5388, -27.5694)
  line L309 (7.8388, -25.8694) -> (3.5388, -25.8694)
  line L310 (7.8388, -24.8694) -> (7.8388, -25.8694)
  line L311 (3.5388, -24.8694) -> (7.8388, -24.8694)
  line L312 (3.5388, -25.8694) -> (3.5388, -24.8694)
  line L313 (7.8388, -23.1694) -> (3.5388, -23.1694)
  line L314 (7.8388, -22.1694) -> (7.8388, -23.1694)
  line L315 (3.5388, -22.1694) -> (7.8388, -22.1694)
  line L316 (3.5388, -23.1694) -> (3.5388, -22.1694)
  line L317 (7.8388, -20.4694) -> (3.5388, -20.4694)
  line L318 (7.8388, -19.4694) -> (7.8388, -20.4694)
  line L319 (3.5388, -19.4694) -> (7.8388, -19.4694)
  line L320 (3.5388, -20.4694) -> (3.5388, -19.4694)
  line L321 (7.8388, -17.7694) -> (3.5388, -17.7694)
  line L322 (7.8388, -16.7694) -> (7.8388, -17.7694)
  line L323 (3.5388, -16.7694) -> (7.8388, -16.7694)
  line L324 (3.5388, -17.7694) -> (3.5388, -16.7694)
  line L325 (7.8388, -15.0694) -> (3.5388, -15.0694)
  line L326 (7.8388, -14.0694) -> (7.8388, -15.0694)
  line L327 (3.5388, -14.0694) -> (7.8388, -14.0694)
  line L328 (3.5388, -15.0694) -> (3.5388, -14.0694)
  line L329 (7.8388, -12.3694) -> (3.5388, -12.3694)
  line L330 (7.8388, -11.3694) -> (7.8388, -12.3694)
  line L331 (3.5388, -11.3694) -> (7.8388, -11.3694)
  line L332 (3.5388, -12.3694) -> (3.5388, -11.3694)
  line L333 (7.8388, -9.6694) -> (3.5388, -9.6694)
  line L334 (7.8388, -8.6694) -> (7.8388, -9.6694)
  line L335 (3.5388, -8.6694) -> (7.8388, -8.6694)
  line L336 (3.5388, -9.6694) -> (3.5388, -8.6694)
  point P0 (29.127, -43)
  point P1 (22.127, -43)
  point P2 (15.127, -43)
  point P3 (36.127, -40.3571)
  point P4 (29.127, -40.3571)
  point P5 (22.127, -40.3571)
  point P6 (15.127, -40.3571)
  point P7 (36.127, -37.7143)
  point P8 (29.127, -37.7143)
  point P9 (22.127, -37.7143)
  point P10 (15.127, -37.7143)
  point P11 (36.127, -35.0714)
  point P12 (29.127, -35.0714)
  point P13 (22.127, -35.0714)
  point P14 (15.127, -35.0714)
  point P15 (36.127, -32.4286)
  point P16 (29.127, -32.4286)
  point P17 (22.127, -32.4286)
  point P18 (15.127, -32.4286)
  point P19 (36.127, -29.7857)
  point P20 (29.127, -29.7857)
  point P21 (22.127, -29.7857)
  point P22 (15.127, -29.7857)
  point P23 (36.127, -27.1429)
  point P24 (29.127, -27.1429)
  point P25 (22.127, -27.1429)
  point P26 (15.127, -27.1429)
  point P27 (36.127, -24.5)
  point P28 (29.127, -24.5)
  point P29 (22.127, -24.5)
  point P30 (15.127, -24.5)
  point P31 (36.127, -21.8571)
  point P32 (29.127, -21.8571)
  point P33 (22.127, -21.8571)
  point P34 (15.127, -21.8571)
  point P35 (36.127, -19.2143)
  point P36 (29.127, -19.2143)
  point P37 (22.127, -19.2143)
  point P38 (15.127, -19.2143)
  point P39 (36.127, -16.5714)
  point P40 (29.127, -16.5714)
  point P41 (22.127, -16.5714)
  point P42 (15.127, -16.5714)
  point P43 (36.127, -13.9286)
  point P44 (29.127, -13.9286)
  point P45 (22.127, -13.9286)
  point P46 (15.127, -13.9286)
  point P47 (36.127, -11.2857)
  point P48 (29.127, -11.2857)
  point P49 (22.127, -11.2857)
  point P50 (15.127, -11.2857)
  point P51 (36.127, -8.6429)
  point P52 (29.127, -8.6429)
  point P53 (22.127, -8.6429)
  point P54 (15.127, -8.6429)
  point P55 (36.127, -6)
  point P56 (29.127, -6)
  point P57 (22.127, -6)
  point P58 (15.127, -6)
  point P59 (36.127, -32.3714)
  point P60 (36.127, -29.6714)
  point P61 (36.127, -26.9714)
  point P62 (36.127, -24.2714)
  point P63 (36.127, -21.5714)
  point P64 (36.127, -18.8714)
  point P65 (36.127, -16.1714)
  point P66 (36.127, -13.4714)
  point P67 (36.127, -10.7714)
  point P68 (36.127, -8.0714)
  dimension "d58" = 6
  dimension "d59" = 6
  dimension "d60" = 6
  dimension "d61" = 6
  dimension "d62" = 8
  dimension "d63" = 8
  dimension "d64" = 8
  dimension "d65" = 8
  dimension "d66" = 3
  dimension "d67" = 3
  dimension "d68" = 3
  dimension "d69" = 3
  dimension "d70" = 5
  dimension "d71" = 1
  dimension "d74" = -21
  dimension "d75" = 37
  dimension "d78" = 0
  dimension "d79" = 27
  dimension "d80" = 4.3
  dimension "d81" = 1
  dimension "d84" = 0
  dimension "d85" = 27
  constraint concentric A2 A4
  constraint concentric A1 A5
  constraint concentric A3 A6
  constraint concentric A0 A7
  constraint concentric A4 A13
  constraint concentric A5 A11
  constraint concentric A6 A8
  constraint concentric A7 A9
  constraint parallel L2 L4
  constraint horizontal L5
  constraint parallel L0 L6
  constraint perpendicular L4 L7
  constraint concentric A9 A10
  constraint concentric A11 A12
  constraint concentric A13 A14
  constraint horizontal L8
  constraint vertical L9
  constraint horizontal L10
  constraint vertical L11
  constraint horizontal L248
  constraint vertical L249
  constraint horizontal L250
  constraint vertical L251
  constraint perpendicular L248 L252
  constraint horizontal L293
  constraint vertical L294
  constraint horizontal L295
  constraint vertical L296
  measures "d58" diameter of A4
  measures "d59" diameter of A5
  measures "d60" diameter of A6
  measures "d61" diameter of A7
  measures "d62" diameter of A13
  measures "d63" diameter of A11
  measures "d64" diameter of A8
  measures "d65" diameter of A9
  measures "d66" distance of L2 L4
  measures "d67" distance of L3 L7
  measures "d68" distance of L0 L6
  measures "d69" distance of L1 L5
  measures "d70" distance of L8.start L8.end
  measures "d71" distance of L8.start L10.end
  measures "d80" distance of L293.start L293.end
  measures "d81" distance of L293.start L295.end
extrude "拉伸9" cut sketch "草图9" against normal blind 5 contours L4 L5 L6 L7 A8 A9 A11 A13 bodies 1
extrude "拉伸10" add sketch "草图9" along normal blind 1 contours A4 | A5 | A6 | A7 bodies 1
sketch "草图10" plane through (0, 0, 0) normal (0, -1, 0) x (1, 0, 0)
  line L0 (4, 0) -> (40, 0)
  line L1 (40, 0) -> (40, 30.5)
  line L2 (40, 30.5) -> (4, 30.5)
  line L3 (4, 30.5) -> (4, 0)
  line L4 (10, 22.5) -> (15, 22.5)
  line L5 (15, 22.5) -> (15, 9.5)
  line L6 (15, 9.5) -> (10, 9.5)
  line L7 (10, 9.5) -> (10, 22.5)
  line L8 (20, 22.5) -> (36, 22.5)
  line L9 (36, 22.5) -> (36, 8)
  line L10 (36, 8) -> (20, 8)
  line L11 (20, 8) -> (20, 22.5)
  dimension "d90" = 5
  dimension "d91" = 13
  dimension "d93" = 6
  dimension "d94" = 8
  dimension "d95" = 16
  dimension "d96" = 14.5
  dimension "d97" = 8
  dimension "d98" = 4
  constraint horizontal L4
  constraint vertical L5
  constraint horizontal L6
  constraint vertical L7
  constraint horizontal L8
  constraint vertical L9
  constraint horizontal L10
  constraint vertical L11
  measures "d90" distance of L4.start L4.end
  measures "d91" distance of L4.start L6.end
  measures "d93" distance of L3 L7
  measures "d94" distance of L2 L4
  measures "d95" distance of L8.start L8.end
  measures "d96" distance of L8.start L10.end
  measures "d97" distance of L2 L8
  measures "d98" distance of L1 L9
extrude "拉伸11" cut sketch "草图10" against normal blind 10 contours L4 L5 L6 L7 | L8 L9 L10 L11 bodies 1
sketch "草图11" plane through (0, 46, 0) normal (0, 1, 0) x (-1, 0, 0)
  line L0 (-40, 0) -> (-4, 0)
  line L1 (-4, 0) -> (-4, 30.5)
  line L2 (-4, 30.5) -> (-40, 30.5)
  line L3 (-40, 30.5) -> (-40, 0)
  line L4 (-38, 27.5) -> (-5, 27.5)
  line L5 (-5, 27.5) -> (-5, 4.5)
  line L6 (-5, 4.5) -> (-38, 4.5)
  line L7 (-38, 4.5) -> (-38, 27.5)
  dimension "d101" = 33
  dimension "d102" = 23
  dimension "d103" = 1
  dimension "d104" = 3
  constraint horizontal L4
  constraint vertical L5
  constraint horizontal L6
  constraint vertical L7
  measures "d101" distance of L4.start L4.end
  measures "d102" distance of L4.start L6.end
  measures "d103" distance of L1 L5
  measures "d104" distance of L2 L4
extrude "拉伸12" cut sketch "草图11" against normal blind 1.5 contours L4 L5 L6 L7 bodies 1
sketch "草图12" plane through (0, 44.5, 0) normal (0, 1, 0) x (-1, 0, 0)
  line L0 (-38, 4.5) -> (-5, 4.5)
  line L1 (-5, 4.5) -> (-5, 27.5)
  line L2 (-5, 27.5) -> (-38, 27.5)
  line L3 (-38, 27.5) -> (-38, 4.5)
  circle A0 centre (-31, 22.5) radius 2.5
  line L4 (-38, 27.5) -> (-5, 27.5)
  line L5 (-38, 4.5) -> (-38, 27.5)
  line L6 (-21, 24.5) -> (-8, 24.5)
  line L7 (-8, 24.5) -> (-8, 18.5)
  line L8 (-8, 18.5) -> (-21, 18.5)
  line L9 (-21, 18.5) -> (-21, 24.5)
  line L10 (-5, 27.5) -> (-5, 4.5)
  line L11 (-21, 10.5) -> (-9, 10.5)
  line L12 (-9, 10.5) -> (-9, 8.5)
  line L13 (-9, 8.5) -> (-21, 8.5)
  line L14 (-21, 8.5) -> (-21, 10.5)
  line L15 (-5, 4.5) -> (-38, 4.5)
  line L16 (-36, 11.5) -> (-28, 11.5)
  line L17 (-28, 11.5) -> (-28, 9.5)
  line L18 (-28, 9.5) -> (-29, 8.5)
  line L19 (-29, 8.5) -> (-35, 8.5)
  line L20 (-36, 11.5) -> (-36, 9.5)
  line L21 (-36, 9.5) -> (-35, 8.5)
  dimension "d107" = 5
  dimension "d108" = 5
  dimension "d109" = 7
  dimension "d110" = 13
  dimension "d111" = 6
  dimension "d112" = 3
  dimension "d113" = 3
  dimension "d114" = 12
  dimension "d115" = 2
  dimension "d116" = 4
  dimension "d117" = 4
  dimension "d118" = 8
  dimension "d119" = 2
  dimension "d120" = 4
  dimension "d121" = 2
  constraint horizontal L6
  constraint vertical L7
  constraint horizontal L8
  constraint vertical L9
  constraint horizontal L11
  constraint vertical L12
  constraint horizontal L13
  constraint vertical L14
  constraint horizontal L16
  constraint perpendicular L16 L17
  constraint perpendicular L17 L19
  constraint perpendicular L16 L20
  measures "d107" diameter of A0
  measures "d108" distance of A0.centre L4
  measures "d109" distance of A0.centre L5
  measures "d110" distance of L6.start L6.end
  measures "d111" distance of L6.start L8.end
  measures "d112" distance of L4 L6
  measures "d113" distance of L7 L10
  measures "d114" distance of L11.start L11.end
  measures "d115" distance of L11.start L13.end
  measures "d116" distance of L13 L15
  measures "d117" distance of L10 L12
  measures "d118" distance of L16.start L16.end
  measures "d119" distance of L16.end L17.end
  measures "d120" distance of L15 L19
  measures "d121" distance of L5 L20
extrude "拉伸13" cut sketch "草图12" against normal blind 10 contours L6 L7 L8 L9 bodies 1
extrude "拉伸14" cut sketch "草图12" against normal blind 10 contours A0 | L11 L12 L13 L14 | L16 L17 L18 L19 L20 L21 bodies 1
combine "合并1" operation add target body 1 tool bodies 2 3 4 5
copy_body "实体->零部件1" bodies 1 removing the originals makes body 6 in component "NanoPi"
component "NanoPi" placed x (1, 0, 0) y (0, 1, 0) z (0, 0, 1) at (0, 0, 0)
